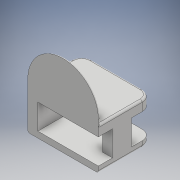
# Autodesk Inventor part: Base
Saved by Autodesk Inventor 2018 (Build 220112000, 112)
## iProperties
Created: 2021-08-18
Part Number: Base
Material: Generic
Document SubType Name: Modeling
Designer: dangl
Density: 1 g/cm^3
Appearance: Default
Author: dangl
Autodesk Inventor part; units mm, degrees
ref_plane "YZ Plane" through (0, 0, 0) normal (1, 0, 0) x (0, 1, 0)
ref_plane "XZ Plane" through (0, 0, 0) normal (0, 1, 0) x (-1, 0, 0)
ref_plane "XY Plane" through (0, 0, 0) normal (0, 0, 1) x (1, 0, 0)
sketch "Sketch1" plane through (0, 0, 0) normal (0, 1, 0) x (-1, 0, 0)
  arc A0 (17.5, 0) -> (-17.5, 0) centre (0, 0) ccw
  line L0 (17.5, 0) -> (-17.5, 0)
  line L1 (-17.5, 0) -> (-17.5, -23)
  line L2 (-17.5, -23) -> (17.5, -23)
  line L3 (17.5, -23) -> (17.5, 0)
  line L4 (12.5, -20) -> (-12.5, -20)
  line L5 (-12.5, -20) -> (-12.5, -7.5)
  line L6 (-12.5, -7.5) -> (12.5, -7.5)
  line L7 (12.5, -7.5) -> (12.5, -20)
  line L8 (17.5, -2.5) -> (-17.5, -2.5)
  line L9 (-12.5, -20) -> (-17.5, -20)
  line L10 (12.5, -20) -> (17.5, -20)
  line L11 (12.5, -7.5) -> (17.5, -7.5)
  line L12 (-12.5, -7.5) -> (-17.5, -7.5)
  dimension "d0" = 35
  dimension "d1" = 35
  dimension "d2" = 23
  dimension "d3" = 25
  dimension "d4" = 12.5
  dimension "d5" = 12.5
  dimension "d6" = 3
  dimension "d7" = 5
  constraints: 26 end point, 8 point on line, 5 perpendicular, 4 parallel, 2 horizontal, 2 point on circle, 1 centre point, 1 coincident
  measures "d0" distance of L1.end L2.end
  measures "d1" diameter of A0
  measures "d2" distance of L0.end L1.end
  measures "d3" distance of L4.start L4.end
  measures "d4" distance of L4.end L5.end
  measures "d5" distance from line of point (0, 0) L7
  measures "d6" distance between parallel lines of L2 L4
  measures "d7" distance between parallel lines of L6 L8
extrude "Extrusion1" add sketch "Sketch1" along normal blind 1 contours L0 A0 | L3 L8 L1 L0
extrude "Extrusion2" add sketch "Sketch1" along normal blind 16.5 contours L3 L10 L7 L11 | L12 L5 L9 L1
extrude "Extrusion3" add sketch "Sketch1" along normal blind 26.7 contours L3 L11 L6 L12 L1 L8 | L3 L2 L1 L9 L4 L10
extrude "Extrusion4" cut sketch "Sketch1" along normal blind 7 contours L12 L5 L9 L1
fillet "Fillet1" radius 1 3 edges at (17.5, 1, -1.25) (-17.5, 1, -1.25) (0, 1, 17.5)
fillet "Fillet2" radius 5 4 edges at (17.5, 26.7, -5) (17.5, 26.7, -21.5) (-17.5, 26.7, -21.5) (-17.5, 26.7, -5)
fillet "Fillet3" radius 1 12 edges at (16.0355, 25.2355, -2.5) (17.5, 11.35, -2.5) (17.5, 0.5001, -2.5) (-16.0355, 25.2355, -2.5) (-17.5, 0.5001, -2.5) (-17.5, 11.35, -2.5) (0, 26.7, -2.5) (0, 26.7, -23) (-16.0355, 25.2355, -23) (-17.5, 10.85, -23) (17.5, 10.85, -23) (16.0355, 25.2355, -23)
sketch "Sketch2" plane through (0, 16.5, 0) normal (0, 1, 0) x (1, 0, 0)
  circle A0 centre (-13.83, 13.75) radius 0.5
  circle A1 centre (13.83, 13.75) radius 0.5
  point P0 (0, 0)
  dimension "d19" = 1
  dimension "d20" = 1
  dimension "d21" = 27.66
  dimension "d22" = 13.83
  constraints: 2 centre point
  measures "d19" diameter of A0
  measures "d20" diameter of A1
  measures "d21" distance of A0.centre A1.centre
  measures "d22" horizontal distance of point (0, 0) A0.centre
extrude "Extrusion5" cut sketch "Sketch2" against normal blind 7
equation "\"d0\" = d1"
equation "\"d5\" = 0.5 * d3"
equation "\"d20\" = d19"
equation "\"d22\" = 0.5 * d21"
body "Solid1"
